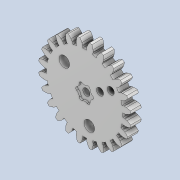
# Autodesk Inventor part: m2z24
Saved by Autodesk Inventor 2020.4 (Build 244396000, 396)
## iProperties
Created: 2021-04-23
Part Number: m2z24
Material: アルミニウム 2014-T4
Document SubType Name: Modeling
Designer: happy
Density: 2.8 g/cm^3
Appearance: サテン
Author: happy
Autodesk Inventor part; units mm, degrees
ref_plane "YZ Plane" through (0, 0, 0) normal (1, 0, 0) x (0, 1, 0)
ref_plane "XZ Plane" through (0, 0, 0) normal (0, 1, 0) x (-1, 0, 0)
ref_plane "XY Plane" through (0, 0, 0) normal (0, 0, 1) x (1, 0, 0)
sketch "スケッチ1" plane through (0, 0, 0) normal (0, 0, 1) x (1, 0, 0)
  arc A0 (149.6906, 127.8379) -> (149.6395, 127.5239) centre (151.8502, 127.3259) ccw
  arc A1 (150.0513, 128.9073) -> (149.6906, 127.8379) centre (155.6312, 126.4296) ccw
  arc A2 (151.183, 130.8613) -> (150.0513, 128.9073) centre (159.7055, 124.6205) ccw
  arc A3 (143.7391, 127.3679) -> (143.7711, 127.0514) centre (145.9577, 127.4323) ccw
  arc A4 (143.8108, 128.4942) -> (143.7391, 127.3679) centre (149.8418, 127.5451) ccw
  arc A5 (144.3982, 130.6746) -> (143.8108, 128.4942) centre (154.2455, 126.8521) ccw
  arc A6 (138.1122, 125.3735) -> (138.225, 125.0761) centre (140.2385, 126.01) ccw
  arc A7 (137.8899, 126.48) -> (138.1122, 125.3735) centre (143.961, 127.1242) ccw
  arc A8 (137.893, 128.7381) -> (137.8899, 126.48) centre (148.394, 127.5946) ccw
  arc A9 (133.1931, 121.9907) -> (133.3791, 121.7327) centre (135.0822, 123.1558) ccw
  arc A10 (132.692, 123.002) -> (133.1931, 121.9907) centre (138.3896, 125.1956) ccw
  arc A11 (132.1105, 125.184) -> (132.692, 123.002) centre (142.5498, 126.7973) ccw
  arc A12 (129.3172, 117.4501) -> (129.5636, 117.2489) centre (130.8404, 119.0644) ccw
  arc A13 (128.5714, 118.2972) -> (129.3172, 117.4501) centre (133.5071, 121.8907) ccw
  arc A14 (127.445, 120.2543) -> (128.5714, 118.2972) centre (137.111, 124.5146) ccw
  arc A15 (126.7485, 112.061) -> (127.0386, 111.9305) centre (127.802, 114.0146) ccw
  arc A16 (125.8089, 112.6862) -> (126.7485, 112.061) centre (129.6464, 117.4347) ccw
  arc A17 (124.2144, 114.2851) -> (125.8089, 112.6862) centre (132.4484, 120.902) ccw
  arc A18 (125.6622, 106.1907) -> (125.9762, 106.1397) centre (126.1742, 108.3504) ccw
  arc A19 (124.5928, 106.5514) -> (125.6622, 106.1907) centre (127.0705, 112.1314) ccw
  arc A20 (122.6388, 107.6832) -> (124.5928, 106.5514) centre (128.8796, 116.2057) ccw
  arc A21 (126.1322, 100.2393) -> (126.4487, 100.2713) centre (126.0678, 102.4579) ccw
  arc A22 (125.0059, 100.311) -> (126.1322, 100.2393) centre (125.955, 106.342) ccw
  arc A23 (122.8255, 100.8984) -> (125.0059, 100.311) centre (126.648, 110.7457) ccw
  arc A24 (128.1266, 94.6123) -> (128.424, 94.7252) centre (127.4901, 96.7387) ccw
  arc A25 (127.0201, 94.39) -> (128.1266, 94.6123) centre (126.3759, 100.4612) ccw
  arc A26 (124.762, 94.3931) -> (127.0201, 94.39) centre (125.9055, 104.8942) ccw
  arc A27 (131.5094, 89.6933) -> (131.7674, 89.8792) centre (130.3443, 91.5824) ccw
  arc A28 (130.4981, 89.1922) -> (131.5094, 89.6933) centre (128.3045, 94.8897) ccw
  arc A29 (128.3161, 88.6107) -> (130.4981, 89.1922) centre (126.7028, 99.05) ccw
  arc A30 (136.05, 85.8174) -> (136.2512, 86.0638) centre (134.4357, 87.3406) ccw
  arc A31 (135.2029, 85.0716) -> (136.05, 85.8174) centre (131.6094, 90.0073) ccw
  arc A32 (133.2458, 83.9452) -> (135.2029, 85.0716) centre (128.9855, 93.6112) ccw
  arc A33 (141.4391, 83.2487) -> (141.5696, 83.5388) centre (139.4855, 84.3022) ccw
  arc A34 (140.8139, 82.3091) -> (141.4391, 83.2487) centre (136.0654, 86.1465) ccw
  arc A35 (139.215, 80.7146) -> (140.8139, 82.3091) centre (132.5981, 88.9485) ccw
  arc A36 (147.3094, 82.1624) -> (147.3604, 82.4764) centre (145.1497, 82.6744) ccw
  arc A37 (146.9487, 81.093) -> (147.3094, 82.1624) centre (141.3687, 83.5707) ccw
  arc A38 (145.8169, 79.1389) -> (146.9487, 81.093) centre (137.2944, 85.3798) ccw
  arc A39 (153.2608, 82.6324) -> (153.2288, 82.9489) centre (151.0422, 82.568) ccw
  arc A40 (153.1891, 81.5061) -> (153.2608, 82.6324) centre (147.1581, 82.4552) ccw
  arc A41 (152.6017, 79.3257) -> (153.1891, 81.5061) centre (142.7544, 83.1481) ccw
  arc A42 (158.8878, 84.6268) -> (158.7749, 84.9242) centre (156.7614, 83.9903) ccw
  arc A43 (159.1101, 83.5203) -> (158.8878, 84.6268) centre (153.0389, 82.8761) ccw
  arc A44 (159.107, 81.2622) -> (159.1101, 83.5203) centre (148.6059, 82.4057) ccw
  arc A45 (163.8068, 88.0095) -> (163.6209, 88.2676) centre (161.9177, 86.8444) ccw
  arc A46 (164.3079, 86.9983) -> (163.8068, 88.0095) centre (158.6104, 84.8047) ccw
  arc A47 (164.8894, 84.8163) -> (164.3079, 86.9983) centre (154.4501, 83.203) ccw
  arc A48 (167.6827, 92.5502) -> (167.4363, 92.7513) centre (166.1595, 90.9358) ccw
  arc A49 (168.4285, 91.7031) -> (167.6827, 92.5502) centre (163.4928, 88.1096) ccw
  arc A50 (169.5549, 89.7459) -> (168.4285, 91.7031) centre (159.8889, 85.4857) ccw
  arc A51 (170.2514, 97.9393) -> (169.9613, 98.0698) centre (169.1979, 95.9857) ccw
  arc A52 (171.191, 97.3141) -> (170.2514, 97.9393) centre (167.3536, 92.5656) ccw
  arc A53 (172.7855, 95.7151) -> (171.191, 97.3141) centre (164.5516, 89.0983) ccw
  arc A54 (171.3377, 103.8095) -> (171.0237, 103.8606) centre (170.8257, 101.6499) ccw
  arc A55 (172.4071, 103.4488) -> (171.3377, 103.8095) centre (169.9294, 97.8689) ccw
  arc A56 (174.3612, 102.3171) -> (172.4071, 103.4488) centre (168.1203, 93.7946) ccw
  arc A57 (170.8677, 109.761) -> (170.5512, 109.729) centre (170.9321, 107.5424) ccw
  arc A58 (171.994, 109.6893) -> (170.8677, 109.761) centre (171.0449, 103.6583) ccw
  arc A59 (174.1744, 109.1019) -> (171.994, 109.6893) centre (170.352, 99.2546) ccw
  arc A60 (168.8733, 115.3879) -> (168.5759, 115.2751) centre (169.5098, 113.2616) ccw
  arc A61 (169.9798, 115.6102) -> (168.8733, 115.3879) centre (170.624, 109.5391) ccw
  arc A62 (172.2379, 115.6071) -> (169.9798, 115.6102) centre (171.0944, 105.1061) ccw
  arc A63 (165.4906, 120.307) -> (165.2325, 120.121) centre (166.6557, 118.4179) ccw
  arc A64 (166.5018, 120.8081) -> (165.4906, 120.307) centre (168.6954, 115.1105) ccw
  arc A65 (168.6838, 121.3896) -> (166.5018, 120.8081) centre (170.2971, 110.9503) ccw
  arc A66 (160.9499, 124.1829) -> (160.7488, 123.9365) centre (162.5643, 122.6597) ccw
  arc A67 (161.797, 124.9287) -> (160.9499, 124.1829) centre (165.3905, 119.993) ccw
  arc A68 (163.7542, 126.0551) -> (161.797, 124.9287) centre (168.0144, 116.3891) ccw
  arc A69 (155.5608, 126.7516) -> (155.4303, 126.4615) centre (157.5144, 125.6981) ccw
  arc A70 (156.186, 127.6912) -> (155.5608, 126.7516) centre (160.9345, 123.8537) ccw
  arc A71 (157.785, 129.2857) -> (156.186, 127.6912) centre (164.4018, 121.0517) ccw
  arc A72 (147.3604, 127.5239) -> (147.3094, 127.8379) centre (145.1497, 127.3259) ccw
  arc A73 (147.3094, 127.8379) -> (146.9487, 128.9073) centre (141.3687, 126.4296) ccw
  arc A74 (146.9487, 128.9073) -> (145.8169, 130.8613) centre (137.2944, 124.6205) ccw
  arc A75 (141.5696, 126.4615) -> (141.4391, 126.7516) centre (139.4855, 125.6981) ccw
  arc A76 (141.4391, 126.7516) -> (140.8139, 127.6912) centre (136.0654, 123.8537) ccw
  arc A77 (140.8139, 127.6912) -> (139.215, 129.2857) centre (132.5981, 121.0517) ccw
  arc A78 (136.2512, 123.9365) -> (136.05, 124.1829) centre (134.4357, 122.6597) ccw
  arc A79 (136.05, 124.1829) -> (135.2029, 124.9287) centre (131.6094, 119.993) ccw
  arc A80 (135.2029, 124.9287) -> (133.2458, 126.0551) centre (128.9855, 116.3891) ccw
  arc A81 (131.7674, 120.121) -> (131.5094, 120.307) centre (130.3443, 118.4179) ccw
  arc A82 (131.5094, 120.307) -> (130.4981, 120.8081) centre (128.3045, 115.1105) ccw
  arc A83 (130.4981, 120.8081) -> (128.3161, 121.3896) centre (126.7028, 110.9503) ccw
  arc A84 (128.424, 115.2751) -> (128.1266, 115.3879) centre (127.4901, 113.2616) ccw
  arc A85 (128.1266, 115.3879) -> (127.0201, 115.6102) centre (126.3759, 109.5391) ccw
  arc A86 (127.0201, 115.6102) -> (124.762, 115.6071) centre (125.9055, 105.1061) ccw
  arc A87 (126.4487, 109.729) -> (126.1322, 109.761) centre (126.0678, 107.5424) ccw
  arc A88 (126.1322, 109.761) -> (125.0059, 109.6893) centre (125.955, 103.6583) ccw
  arc A89 (125.0059, 109.6893) -> (122.8255, 109.1019) centre (126.648, 99.2546) ccw
  arc A90 (125.9762, 103.8606) -> (125.6622, 103.8095) centre (126.1742, 101.6499) ccw
  arc A91 (125.6622, 103.8095) -> (124.5928, 103.4488) centre (127.0705, 97.8689) ccw
  arc A92 (124.5928, 103.4488) -> (122.6388, 102.3171) centre (128.8796, 93.7946) ccw
  arc A93 (127.0386, 98.0698) -> (126.7485, 97.9393) centre (127.802, 95.9857) ccw
  arc A94 (126.7485, 97.9393) -> (125.8089, 97.3141) centre (129.6464, 92.5656) ccw
  arc A95 (125.8089, 97.3141) -> (124.2144, 95.7151) centre (132.4484, 89.0983) ccw
  arc A96 (129.5636, 92.7513) -> (129.3172, 92.5502) centre (130.8404, 90.9358) ccw
  arc A97 (129.3172, 92.5502) -> (128.5714, 91.7031) centre (133.5071, 88.1096) ccw
  arc A98 (128.5714, 91.7031) -> (127.445, 89.7459) centre (137.111, 85.4857) ccw
  arc A99 (133.3791, 88.2676) -> (133.1931, 88.0095) centre (135.0822, 86.8444) ccw
  arc A100 (133.1931, 88.0095) -> (132.692, 86.9983) centre (138.3896, 84.8047) ccw
  arc A101 (132.692, 86.9983) -> (132.1105, 84.8163) centre (142.5498, 83.203) ccw
  arc A102 (138.225, 84.9242) -> (138.1122, 84.6268) centre (140.2385, 83.9903) ccw
  arc A103 (138.1122, 84.6268) -> (137.8899, 83.5203) centre (143.961, 82.8761) ccw
  arc A104 (137.8899, 83.5203) -> (137.893, 81.2622) centre (148.394, 82.4057) ccw
  arc A105 (143.7711, 82.9489) -> (143.7391, 82.6324) centre (145.9577, 82.568) ccw
  arc A106 (143.7391, 82.6324) -> (143.8108, 81.5061) centre (149.8418, 82.4552) ccw
  arc A107 (143.8108, 81.5061) -> (144.3982, 79.3257) centre (154.2455, 83.1481) ccw
  arc A108 (149.6395, 82.4764) -> (149.6906, 82.1624) centre (151.8502, 82.6744) ccw
  arc A109 (149.6906, 82.1624) -> (150.0513, 81.093) centre (155.6312, 83.5707) ccw
  arc A110 (150.0513, 81.093) -> (151.183, 79.1389) centre (159.7055, 85.3798) ccw
  arc A111 (155.4303, 83.5388) -> (155.5608, 83.2487) centre (157.5144, 84.3022) ccw
  arc A112 (155.5608, 83.2487) -> (156.186, 82.3091) centre (160.9345, 86.1465) ccw
  arc A113 (156.186, 82.3091) -> (157.785, 80.7146) centre (164.4018, 88.9485) ccw
  arc A114 (160.7488, 86.0638) -> (160.9499, 85.8174) centre (162.5643, 87.3406) ccw
  arc A115 (160.9499, 85.8174) -> (161.797, 85.0716) centre (165.3905, 90.0073) ccw
  arc A116 (161.797, 85.0716) -> (163.7542, 83.9452) centre (168.0144, 93.6112) ccw
  arc A117 (165.2325, 89.8792) -> (165.4906, 89.6933) centre (166.6557, 91.5824) ccw
  arc A118 (165.4906, 89.6933) -> (166.5018, 89.1922) centre (168.6954, 94.8897) ccw
  arc A119 (166.5018, 89.1922) -> (168.6838, 88.6107) centre (170.2971, 99.05) ccw
  arc A120 (168.5759, 94.7252) -> (168.8733, 94.6123) centre (169.5098, 96.7387) ccw
  arc A121 (168.8733, 94.6123) -> (169.9798, 94.39) centre (170.624, 100.4612) ccw
  arc A122 (169.9798, 94.39) -> (172.2379, 94.3931) centre (171.0944, 104.8942) ccw
  arc A123 (170.5512, 100.2713) -> (170.8677, 100.2393) centre (170.9321, 102.4579) ccw
  arc A124 (170.8677, 100.2393) -> (171.994, 100.311) centre (171.0449, 106.342) ccw
  arc A125 (171.994, 100.311) -> (174.1744, 100.8984) centre (170.352, 110.7457) ccw
  arc A126 (171.0237, 106.1397) -> (171.3377, 106.1907) centre (170.8257, 108.3504) ccw
  arc A127 (171.3377, 106.1907) -> (172.4071, 106.5514) centre (169.9294, 112.1314) ccw
  arc A128 (172.4071, 106.5514) -> (174.3612, 107.6832) centre (168.1203, 116.2057) ccw
  arc A129 (169.9613, 111.9305) -> (170.2514, 112.061) centre (169.1979, 114.0146) ccw
  arc A130 (170.2514, 112.061) -> (171.191, 112.6862) centre (167.3536, 117.4347) ccw
  arc A131 (171.191, 112.6862) -> (172.7855, 114.2851) centre (164.5516, 120.902) ccw
  arc A132 (167.4363, 117.2489) -> (167.6827, 117.4501) centre (166.1595, 119.0644) ccw
  arc A133 (167.6827, 117.4501) -> (168.4285, 118.2972) centre (163.4928, 121.8907) ccw
  arc A134 (168.4285, 118.2972) -> (169.5549, 120.2543) centre (159.8889, 124.5146) ccw
  arc A135 (163.6209, 121.7327) -> (163.8068, 121.9907) centre (161.9177, 123.1558) ccw
  arc A136 (163.8068, 121.9907) -> (164.3079, 123.002) centre (158.6104, 125.1956) ccw
  arc A137 (164.3079, 123.002) -> (164.8894, 125.184) centre (154.4501, 126.7973) ccw
  arc A138 (158.7749, 125.0761) -> (158.8878, 125.3735) centre (156.7614, 126.01) ccw
  arc A139 (158.8878, 125.3735) -> (159.1101, 126.48) centre (153.0389, 127.1242) ccw
  arc A140 (159.1101, 126.48) -> (159.107, 128.7381) centre (148.6059, 127.5946) ccw
  arc A141 (153.2288, 127.0514) -> (153.2608, 127.3679) centre (151.0422, 127.4323) ccw
  arc A142 (153.2608, 127.3679) -> (153.1891, 128.4942) centre (147.1581, 127.5451) ccw
  arc A143 (153.1891, 128.4942) -> (152.6017, 130.6746) centre (142.7544, 126.8521) ccw
  arc A144 (149.5864, 126.4727) -> (147.4136, 126.4727) centre (148.5, 105.0001) ccw
  arc A145 (143.9918, 126.0222) -> (141.8931, 125.4598) centre (148.5, 105.0001) ccw
  arc A146 (138.7045, 124.1391) -> (136.8228, 123.0527) centre (148.5, 105.0001) ccw
  arc A147 (134.0848, 120.9517) -> (132.5484, 119.4153) centre (148.5, 105.0001) ccw
  arc A148 (130.4474, 116.6773) -> (129.361, 114.7956) centre (148.5, 105.0001) ccw
  arc A149 (128.0403, 111.607) -> (127.4779, 109.5083) centre (148.5, 105.0001) ccw
  arc A150 (127.0274, 106.0865) -> (127.0274, 103.9137) centre (148.5, 105.0001) ccw
  arc A151 (127.4779, 100.492) -> (128.0403, 98.3933) centre (148.5, 105.0001) ccw
  arc A152 (129.361, 95.2047) -> (130.4474, 93.323) centre (148.5, 105.0001) ccw
  arc A153 (132.5484, 90.585) -> (134.0848, 89.0486) centre (148.5, 105.0001) ccw
  arc A154 (136.8228, 86.9476) -> (138.7045, 85.8612) centre (148.5, 105.0001) ccw
  arc A155 (141.8931, 84.5404) -> (143.9918, 83.9781) centre (148.5, 105.0001) ccw
  arc A156 (147.4136, 83.5276) -> (149.5864, 83.5276) centre (148.5, 105.0001) ccw
  arc A157 (153.0081, 83.9781) -> (155.1068, 84.5404) centre (148.5, 105.0001) ccw
  arc A158 (158.2954, 85.8612) -> (160.1771, 86.9476) centre (148.5, 105.0001) ccw
  arc A159 (162.9151, 89.0486) -> (164.4515, 90.585) centre (148.5, 105.0001) ccw
  arc A160 (166.5525, 93.323) -> (167.6389, 95.2047) centre (148.5, 105.0001) ccw
  arc A161 (168.9597, 98.3933) -> (169.522, 100.492) centre (148.5, 105.0001) ccw
  arc A162 (169.9725, 103.9137) -> (169.9725, 106.0865) centre (148.5, 105.0001) ccw
  arc A163 (169.522, 109.5083) -> (168.9597, 111.607) centre (148.5, 105.0001) ccw
  arc A164 (167.6389, 114.7956) -> (166.5525, 116.6773) centre (148.5, 105.0001) ccw
  arc A165 (164.4515, 119.4153) -> (162.9151, 120.9517) centre (148.5, 105.0001) ccw
  arc A166 (160.1771, 123.0527) -> (158.2954, 124.1391) centre (148.5, 105.0001) ccw
  arc A167 (155.1068, 125.4598) -> (153.0081, 126.0222) centre (148.5, 105.0001) ccw
  arc A168 (145.8169, 130.8613) -> (144.3982, 130.6746) centre (148.5, 105.0001) ccw
  arc A169 (139.215, 129.2857) -> (137.893, 128.7381) centre (148.5, 105.0001) ccw
  arc A170 (133.2458, 126.0551) -> (132.1105, 125.184) centre (148.5, 105.0001) ccw
  arc A171 (128.3161, 121.3896) -> (127.445, 120.2543) centre (148.5, 105.0001) ccw
  arc A172 (124.762, 115.6071) -> (124.2144, 114.2851) centre (148.5, 105.0001) ccw
  arc A173 (122.8255, 109.1019) -> (122.6388, 107.6832) centre (148.5, 105.0001) ccw
  arc A174 (122.6388, 102.3171) -> (122.8255, 100.8984) centre (148.5, 105.0001) ccw
  arc A175 (124.2144, 95.7151) -> (124.762, 94.3931) centre (148.5, 105.0001) ccw
  arc A176 (127.445, 89.7459) -> (128.3161, 88.6107) centre (148.5, 105.0001) ccw
  arc A177 (132.1105, 84.8163) -> (133.2458, 83.9452) centre (148.5, 105.0001) ccw
  arc A178 (137.893, 81.2622) -> (139.215, 80.7146) centre (148.5, 105.0001) ccw
  arc A179 (144.3982, 79.3257) -> (145.8169, 79.1389) centre (148.5, 105.0001) ccw
  arc A180 (151.183, 79.1389) -> (152.6017, 79.3257) centre (148.5, 105.0001) ccw
  arc A181 (157.785, 80.7146) -> (159.107, 81.2622) centre (148.5, 105.0001) ccw
  arc A182 (163.7542, 83.9452) -> (164.8894, 84.8163) centre (148.5, 105.0001) ccw
  arc A183 (168.6838, 88.6107) -> (169.5549, 89.7459) centre (148.5, 105.0001) ccw
  arc A184 (172.2379, 94.3931) -> (172.7855, 95.7151) centre (148.5, 105.0001) ccw
  arc A185 (174.1744, 100.8984) -> (174.3612, 102.3171) centre (148.5, 105.0001) ccw
  arc A186 (174.3612, 107.6832) -> (174.1744, 109.1019) centre (148.5, 105.0001) ccw
  arc A187 (172.7855, 114.2851) -> (172.2379, 115.6071) centre (148.5, 105.0001) ccw
  arc A188 (169.5549, 120.2543) -> (168.6838, 121.3896) centre (148.5, 105.0001) ccw
  arc A189 (164.8894, 125.184) -> (163.7542, 126.0551) centre (148.5, 105.0001) ccw
  arc A190 (159.107, 128.7381) -> (157.785, 129.2857) centre (148.5, 105.0001) ccw
  arc A191 (152.6017, 130.6746) -> (151.183, 130.8613) centre (148.5, 105.0001) ccw
  line L0 (149.5864, 126.4727) -> (149.6395, 127.5239)
  line L1 (143.9918, 126.0222) -> (143.7711, 127.0514)
  line L2 (138.7045, 124.1391) -> (138.225, 125.0761)
  line L3 (134.0848, 120.9517) -> (133.3791, 121.7327)
  line L4 (130.4474, 116.6773) -> (129.5636, 117.2489)
  line L5 (128.0403, 111.607) -> (127.0386, 111.9305)
  line L6 (127.0274, 106.0865) -> (125.9762, 106.1397)
  line L7 (127.4779, 100.492) -> (126.4487, 100.2713)
  line L8 (129.361, 95.2047) -> (128.424, 94.7252)
  line L9 (132.5484, 90.585) -> (131.7674, 89.8792)
  line L10 (136.8228, 86.9476) -> (136.2512, 86.0638)
  line L11 (141.8931, 84.5404) -> (141.5696, 83.5388)
  line L12 (147.4136, 83.5276) -> (147.3604, 82.4764)
  line L13 (153.0081, 83.9781) -> (153.2288, 82.9489)
  line L14 (158.2954, 85.8612) -> (158.7749, 84.9242)
  line L15 (162.9151, 89.0486) -> (163.6209, 88.2676)
  line L16 (166.5525, 93.323) -> (167.4363, 92.7513)
  line L17 (168.9597, 98.3933) -> (169.9613, 98.0698)
  line L18 (169.9725, 103.9137) -> (171.0237, 103.8606)
  line L19 (169.522, 109.5083) -> (170.5512, 109.729)
  line L20 (167.6389, 114.7956) -> (168.5759, 115.2751)
  line L21 (164.4515, 119.4153) -> (165.2325, 120.121)
  line L22 (160.1771, 123.0527) -> (160.7488, 123.9365)
  line L23 (155.1068, 125.4598) -> (155.4303, 126.4615)
  line L24 (147.4136, 126.4727) -> (147.3604, 127.5239)
  line L25 (141.8931, 125.4598) -> (141.5696, 126.4615)
  line L26 (136.8228, 123.0527) -> (136.2512, 123.9365)
  line L27 (132.5484, 119.4153) -> (131.7674, 120.121)
  line L28 (129.361, 114.7956) -> (128.424, 115.2751)
  line L29 (127.4779, 109.5083) -> (126.4487, 109.729)
  line L30 (127.0274, 103.9137) -> (125.9762, 103.8606)
  line L31 (128.0403, 98.3933) -> (127.0386, 98.0698)
  line L32 (130.4474, 93.323) -> (129.5636, 92.7513)
  line L33 (134.0848, 89.0486) -> (133.3791, 88.2676)
  line L34 (138.7045, 85.8612) -> (138.225, 84.9242)
  line L35 (143.9918, 83.9781) -> (143.7711, 82.9489)
  line L36 (149.5864, 83.5276) -> (149.6395, 82.4764)
  line L37 (155.1068, 84.5404) -> (155.4303, 83.5388)
  line L38 (160.1771, 86.9476) -> (160.7488, 86.0638)
  line L39 (164.4515, 90.585) -> (165.2325, 89.8792)
  line L40 (167.6389, 95.2047) -> (168.5759, 94.7252)
  line L41 (169.522, 100.492) -> (170.5512, 100.2713)
  line L42 (169.9725, 106.0865) -> (171.0237, 106.1397)
  line L43 (168.9597, 111.607) -> (169.9613, 111.9305)
  line L44 (166.5525, 116.6773) -> (167.4363, 117.2489)
  line L45 (162.9151, 120.9517) -> (163.6209, 121.7327)
  line L46 (158.2954, 124.1391) -> (158.7749, 125.0761)
  line L47 (153.0081, 126.0222) -> (153.2288, 127.0514)
  line L48 (120.5, 105) -> (176.5, 105) construction
  line L49 (148.5, 77) -> (148.5, 133) construction
  line L50 (194.5, 131.0001) -> (264.5, 131.0001)
  line L51 (194.5, 123.0001) -> (264.5, 123.0001)
  line L52 (194.5, 115.0001) -> (264.5, 115.0001)
  line L53 (194.5, 107.0001) -> (264.5, 107.0001)
  line L54 (194.5, 99.0001) -> (264.5, 99.0001)
  line L55 (194.5, 91.0001) -> (264.5, 91.0001)
  line L56 (194.5, 83.0001) -> (264.5, 83.0001)
  line L57 (194.5, 75.0001) -> (264.5, 75.0001)
  line L58 (194.5, 67.0001) -> (264.5, 67.0001)
  line L59 (194.5, 59.0001) -> (264.5, 59.0001)
  line L60 (194.5, 51.0001) -> (264.5, 51.0001)
  line L61 (194.5, 43.0001) -> (264.5, 43.0001)
  line L62 (194.5, 35.0001) -> (264.5, 35.0001)
  line L63 (194.5, 131.0001) -> (194.5, 35.0001)
  line L64 (264.5, 131.0001) -> (264.5, 35.0001)
  line L65 (229.5, 123.0001) -> (229.5, 35.0001)
  circle A192 centre (148.5, 105.0001) radius 5 construction
  line L66 (148.5, 105.0001) -> (178.8109, 122.5001) construction
  circle A193 centre (163.2224, 113.5001) radius 2
  circle A194 centre (157.1602, 110.0001) radius 2
  line L67 (143.5, 105) -> (145.9998, 109.3302) construction
  line L68 (145.9998, 109.3302) -> (150.9998, 109.3303) construction
  line L69 (150.9998, 109.3303) -> (153.5, 105.0003) construction
  line L70 (153.5, 105.0003) -> (151.0001, 100.6701) construction
  line L71 (151.0001, 100.6701) -> (146.0001, 100.6699) construction
  line L72 (146.0001, 100.6699) -> (143.5, 105) construction
  arc A195 (144.0249, 105.9093) -> (144.025, 104.0907) centre (144.55, 105) ccw
  arc A196 (145.4751, 101.5793) -> (147.0501, 100.67) centre (146.5251, 101.5793) ccw
  arc A197 (149.9501, 100.6701) -> (151.5251, 101.5794) centre (150.4751, 101.5794) ccw
  arc A198 (152.975, 104.0909) -> (152.9749, 105.9096) centre (152.45, 105.0002) ccw
  arc A199 (151.5249, 108.421) -> (149.9498, 109.3303) centre (150.4749, 108.421) ccw
  arc A200 (147.0498, 109.3302) -> (145.4749, 108.4209) centre (146.5249, 108.4209) ccw
  arc A201 (144.0249, 105.9093) -> (145.4749, 108.4209) centre (142.5749, 108.4208) ccw
  arc A202 (145.4751, 101.5793) -> (144.025, 104.0907) centre (142.5751, 101.5792) ccw
  arc A203 (149.9501, 100.6701) -> (147.0501, 100.67) centre (148.5002, 98.1585) ccw
  arc A204 (152.975, 104.0909) -> (151.5251, 101.5794) centre (154.4251, 101.5795) ccw
  arc A205 (151.5249, 108.421) -> (152.9749, 105.9096) centre (154.4249, 108.4211) ccw
  arc A206 (147.0498, 109.3302) -> (149.9498, 109.3303) centre (148.4998, 111.8417) ccw
  circle A207 centre (148.5, 105.0001) radius 2
  point P0 (0, 0)
  point P1 (200.5, 125)
  point P2 (203, 117)
  point P3 (203, 109)
  point P4 (200.5, 101)
  point P5 (203, 93)
  point P6 (198, 85)
  point P7 (200.5, 77)
  point P8 (200.5, 69)
  point P9 (200.5, 61)
  point P10 (203, 53)
  point P11 (203, 45)
  point P12 (200.5, 37)
  point P13 (230.5, 117)
  point P14 (245.5, 109)
  point P15 (246.75, 101)
  point P16 (243, 93)
  point P17 (245.5, 85)
  point P18 (239.25, 77)
  point P19 (245.5, 69)
  point P20 (245.5, 61)
  point P21 (240.5, 53)
  point P22 (248, 45)
  point P23 (248, 37)
  point P24 (149.5, 146.5)
  point P25 (149.5, 140.5)
  point P26 (165.6875, 146.5)
  point P27 (167.8125, 140.5)
  point P28 (146.0001, 100.6699)
  point P29 (153.5, 105.0003)
  point P30 (150.9998, 109.3303)
  point P31 (145.9998, 109.3302)
  point P32 (149.9498, 109.3303)
  point P33 (151.5249, 108.421)
  point P34 (152.9749, 105.9096)
  point P35 (149.9501, 100.6701)
  point P36 (147.0501, 100.67)
  point P37 (145.4751, 101.5793)
  point P38 (144.025, 104.0907)
  dimension "d0" = 10
  dimension "d1" = 35
  dimension "d2" = 30
  dimension "d3" = 4
  dimension "d4" = 4
  dimension "d5" = 10
  dimension "d6" = 7
  dimension "d11" = 360
  dimension "d15" = 360
  dimension "d17" = 1.05
  dimension "d18" = 4
  constraints: 318 point on circle, 159 centre point, 142 end point, 141 equal radius, 98 tangent, 37 parallel, 27 horizontal, 14 perpendicular, 5 point on line, 2 coincident, 2 horizontal alignment, 2 midpoint, 2 vertical alignment, 1 vertical, 847 other
  measures "d1" distance of L66.start L66.end
  measures "d2" angle of L48 L66
  measures "d3" diameter of A193
  measures "d4" diameter of A194
  measures "d5" distance of L66.start A194.centre
  measures "d6" distance of A193.centre A194.centre
  measures "d17" radius of A195
  measures "d18" diameter of A207
extrude "押し出し1" add sketch "スケッチ1" along normal blind 6 contours A1 A2 A191 A143 A142 A141 L47 A167 L23 A69 A70 A71 A190 A140 A139 A138 L46 A166 L22 A66 A67 A68 A189 A137 A136 A135 L45 A165 L21 A63 A64 A65 A188 A134 A133 A132 L44 A164 L20 A60 A61 A62 A187 A131 A130 A129 L43 A163 L19 A57 A58 A59 A186 A128 A127 A126 L42 A162 L18 A54 A55 A56 A185 A125 A124 A123 L41 A161 L17 A51 A52 A53 A184 A122 A121 A120 L40 A160 L16 A48 A49 A50 A183 A119 A118 A117 L39 A159 L15 A45 A46 A47 A182 A116 A115 A114 L38 A158 L14 A42 A43 A44 A181 A113 A112 A111 L37 A157 L13 A39 A40 A41 A180 A110 A109 A108 L36 A156 L12 A36 A37 A38 A179 A107 A106 A105 L35 A155 L11 A33 A34 A35 A178 A104 A103 A102 L34 A154 L10 A30 A31 A32 A177 A101 A100 A99 L33 A153 L9 A27 A28 A29 A176 A98 A97 A96 L32 A152 L8 A24 A25 A26 A175 A95 A94 A93 L31 A151 L7 A21 A22 A23 A174 A92 A91 A90 L30 A150 L6 A18 A19 A20 A173 A89 A88 A87 L29 A149 L5 A15 A16 A17 A172 A86 A85 A84 L28 A148 L4 A12 A13 A14 A171 A83 A82 A81 L27 A147 L3 A9 A10 A11 A170 A80 A79 A78 L26 A146 L2 A6 A7 A8 A169 A77 A76 A75 L25 A145 L1 A3 A4 A5 A168 A74 A73 A72 L24 A144 L0 A0
extrude "押し出し2" add sketch "スケッチ1" along normal blind 5 contours A201 A200 A206 A199 A205 A198 A204 A197 A203 A196 A202 A195
chamfer "面取り1" distance 1.5 angle 45 2 edges at (155.1602, 110.0001, 0) (161.2224, 113.5001, 0)
sketch "スケッチ2" plane through (0, 0, 0) normal (0, 0, -1) x (-1, 0, 0)
  circle A0 centre (-137.0093, 114.642) radius 3
  circle A1 centre (-148.5, 105.0001) radius 2 projected
  circle A2 centre (-148.5, 105.0001) radius 2 projected
  line L0 (-137.0093, 114.642) -> (-148.5, 105.0001)
  line L1 (-148.5, 77) -> (-148.5, 133) construction
  line L2 (-148.5, 105.0001) -> (-178.8109, 122.5001) construction
  circle A3 centre (-151.1047, 90.2279) radius 3
  line L3 (-151.1047, 90.2279) -> (-148.5, 105)
  point P0 (0, 0)
  dimension "d24" = 6
  dimension "d25" = 15
  dimension "d27" = 110
  dimension "d30" = 6
  dimension "d31" = 110
  constraints: 4 end point, 2 centre point, 1 equal length, 1 midpoint
  measures "d24" diameter of A0
  measures "d25" distance of L0.start A1.centre
  measures "d27" angle of L0 L2
  measures "d30" diameter of A3
  measures "d31" angle of L2 L3
extrude "押し出し3" cut sketch "スケッチ2" against normal blind 10 contours A0 | A3
equation "\"d31\" = d27"
